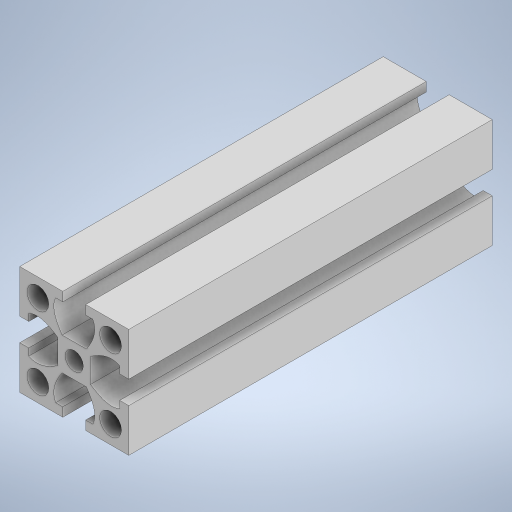
# Autodesk Inventor part: 3030 Aluminium Profile 530mm
Saved by Autodesk Inventor 2023.2 (Build 272271030, 271C)
## iProperties
Created: 2022-10-18
Part Number: 3030 Aluminium Profile 530mm
Material: 일반
Document SubType Name: Modeling
Designer: 박동준
Density: 1 g/cm^3
Appearance: 기본값
Sheet Metal Rule: Default_mm
품번: 9
Author: 박동준
Autodesk Inventor part; units mm, degrees
ref_plane "YZ Plane" through (0, 0, 0) normal (1, 0, 0) x (0, 1, 0)
ref_plane "XZ Plane" through (0, 0, 0) normal (0, 1, 0) x (-1, 0, 0)
ref_plane "XY Plane" through (0, 0, 0) normal (0, 0, 1) x (1, 0, 0)
sketch "스케치1" plane through (0, 0, 0) normal (0, 0, 1) x (1, 0, 0)
  line L0 (3.335, 4.5) -> (0, 4.5)
  spline S0 degree 2 poles (3.335, 4.5) (6.7448, 9.4043) (5.1, 12.5) knots 0 0 0 1 1 1
  line L1 (4.5, 3.335) -> (4.5, 0)
  line L2 (-15, 15) -> (-15, -15)
  line L3 (-15, -15) -> (15, -15)
  line L4 (15, -15) -> (-15, 15) construction
  line L5 (-15, -15) -> (15, 15) construction
  line L6 (15, -3.15) -> (12.5, -3.15)
  line L7 (4.5, -3.335) -> (4.5, 0)
  line L8 (12.5, -3.15) -> (12.5, -5.1)
  spline S1 degree 2 poles (4.5, -3.335) (9.4043, -6.7448) (12.5, -5.1) knots 0 0 0 1 1 1
  line L9 (15, -15) -> (15, 15)
  circle A0 centre (10, -10) radius 3
  line L10 (15, 3.15) -> (12.5, 3.15)
  circle A1 centre (10, 10) radius 3
  spline S2 degree 2 poles (4.5, 3.335) (9.4043, 6.7448) (12.5, 5.1) knots 0 0 0 1 1 1
  line L11 (3.15, 12.5) -> (5.1, 12.5)
  line L12 (15, 15) -> (-15, 15)
  line L13 (0, 0) -> (0, 15) construction
  line L14 (3.15, 15) -> (3.15, 12.5)
  line L15 (-3.15, 15) -> (-3.15, 12.5)
  line L16 (-3.15, 12.5) -> (-5.1, 12.5)
  line L17 (-3.335, 4.5) -> (0, 4.5)
  spline S3 degree 2 poles (-3.335, 4.5) (-6.7448, 9.4043) (-5.1, 12.5) knots 0 0 0 1 1 1
  line L18 (-4.5, 3.335) -> (-4.5, 0)
  spline S4 degree 2 poles (-4.5, 3.335) (-9.4043, 6.7448) (-12.5, 5.1) knots 0 0 0 1 1 1
  line L19 (-12.5, 3.15) -> (-12.5, 5.1)
  line L20 (-15, 3.15) -> (-12.5, 3.15)
  circle A2 centre (-10, 10) radius 3
  circle A3 centre (0, 0) radius 2.5
  line L21 (-4.5, -3.335) -> (-4.5, 0)
  line L22 (-15, -3.15) -> (-12.5, -3.15)
  line L23 (-12.5, -3.15) -> (-12.5, -5.1)
  spline S5 degree 2 poles (-4.5, -3.335) (-9.4043, -6.7448) (-12.5, -5.1) knots 0 0 0 1 1 1
  line L24 (-3.335, -4.5) -> (0, -4.5)
  circle A4 centre (-10, -10) radius 3
  line L25 (3.335, -4.5) -> (0, -4.5)
  spline S6 degree 2 poles (-3.335, -4.5) (-6.7448, -9.4043) (-5.1, -12.5) knots 0 0 0 1 1 1
  line L26 (-3.15, -12.5) -> (-5.1, -12.5)
  line L27 (-3.15, -15) -> (-3.15, -12.5)
  spline S7 degree 2 poles (3.335, -4.5) (6.7448, -9.4043) (5.1, -12.5) knots 0 0 0 1 1 1
  line L28 (3.15, -12.5) -> (5.1, -12.5)
  line L29 (3.15, -15) -> (3.15, -12.5)
  line L30 (12.5, 3.15) -> (12.5, 5.1)
  point P0 (5.5866, 9.5531)
  point P1 (9.5531, -5.5866)
  point P2 (9.5531, 5.5866)
  point P3 (-5.5866, 9.5531)
  point P4 (-9.5531, 5.5866)
  point P5 (-9.5531, -5.5866)
  point P6 (-5.5866, -9.5531)
  point P7 (5.5866, -9.5531)
  dimension "d2" = 30
  dimension "d3" = 30
  dimension "d4" = 6
  dimension "d5" = 5
  dimension "d6" = 6.3
  dimension "d7" = 10.2
  dimension "d8" = 6.67
  dimension "d9" = 8
  dimension "d10" = 2.5
  dimension "d11" = 360
  dimension "d12" = 20
  constraints: 62 end point, 5 centre point, 5 symmetric about line, 3 midpoint, 3 perpendicular, 3 point on line, 2 coincident, 2 parallel, 1 horizontal, 1 vertical, 109 other
  measures "d2" distance of L4.end L9.end
  measures "d3" distance of L9.end L9.start
  measures "d4" diameter of A1
  measures "d5" diameter of A3
  measures "d6" distance between parallel lines of L14 L15
  measures "d7" distance of L11.end L16.end
  measures "d8" distance of L0.start L17.start
  measures "d9" distance between parallel lines of L0 L11
  measures "d10" distance between parallel lines of L11 L12
  measures "d12" distance of A1.centre A2.centre
extrude "돌출1" add sketch "스케치1" along normal mid plane 100 contours S0 L11 L14 L12 L9 L10 L30 S2 L1 L7 S1 L8 L6 L3 L29 L28 S7 L25 L24 S6 L26 L27 L2 L22 L23 S5 L21 L18 S4 L19 L20 L15 L16 S3 L17 L0
equation "\"TransitionRadius\" = BendRadius"
equation "\"BendRadius\" = 0.5"
